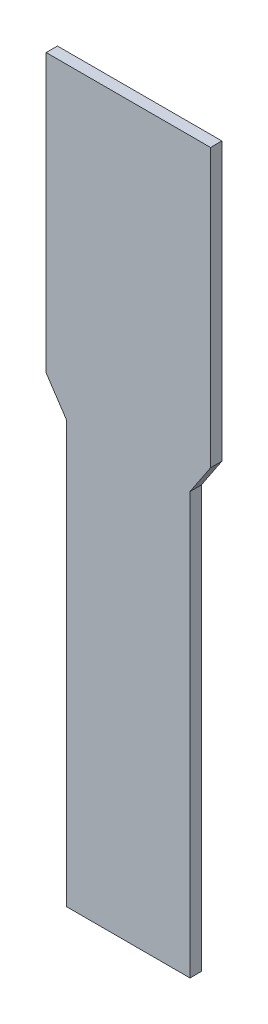
# Autodesk Inventor part: pen_type_cutter_realsize
Saved by Autodesk Inventor 2024 (Build 280153000, 153)
## iProperties
Created: 2025-06-12
Part Number: pen_type_cutter_realsize
Material: 一般
Document SubType Name: Modeling
Designer: 1412z
Density: 1 g/cm^3
Appearance: 既定
Author: 1412z
Autodesk Inventor part; units mm, degrees
ref_plane "YZ Plane" through (0, 0, 0) normal (1, 0, 0) x (0, 1, 0)
ref_plane "XZ Plane" through (0, 0, 0) normal (0, 1, 0) x (-1, 0, 0)
ref_plane "XY Plane" through (0, 0, 0) normal (0, 0, 1) x (1, 0, 0)
sketch "スケッチ1" plane through (0, 0, 0) normal (0, 0, 1) x (1, 0, 0)
  line L0 (-4, 17.75) -> (4, 17.75)
  line L1 (4, 17.75) -> (4, -17.75)
  line L2 (4, -17.75) -> (-4, -17.75)
  line L3 (-4, -17.75) -> (-4, 17.75)
  line L4 (-4, 17.75) -> (4, -17.75) construction
  line L5 (4, 17.75) -> (-4, -17.75) construction
  point P0 (0, 0)
  dimension "d0" = 8
  dimension "d1" = 35.5
  constraints: 12 end point, 2 midpoint, 2 parallel, 1 horizontal, 1 perpendicular
  measures "d0" distance of L1.end L2.end
  measures "d1" distance of L0.end L1.end
extrude "押し出し1" add sketch "スケッチ1" along normal blind 0.55
sketch "スケッチ2" plane through (0, 0, 0.55) normal (0, 0, 1) x (1, 0, 0)
  line L0 (-4, -17.75) -> (4, -17.75) projected
  line L1 (3, -17.75) -> (3, 2.75)
  line L2 (4, -17.75) -> (4, 17.75) projected
  line L3 (3, -17.75) -> (23.5, -17.75) construction
  line L4 (0, -17.75) -> (-3, -17.75)
  line L5 (-3, -17.75) -> (-3, 2.75)
  line L6 (-4, 17.75) -> (-4, -17.75) projected
  line L7 (-4, 4.25) -> (-3, 2.75)
  line L8 (-4, 4.25) -> (-4, -17.75)
  line L9 (-4, -17.75) -> (-3, -17.75)
  line L10 (4, 4.25) -> (3, 2.75)
  line L11 (4, 4.25) -> (4, -17.75)
  line L12 (3, -17.75) -> (4, -17.75)
  point P0 (0, 0)
  dimension "d4" = 20.5
  dimension "d5" = 90
  dimension "d6" = 3
  constraints: 20 end point, 5 point on line, 4 collinear, 2 perpendicular, 1 horizontal, 1 midpoint, 1 parallel
  measures "d4" distance of L1.start L1.end
  measures "d5" angle of L3 L1
  measures "d6" distance of L4.start L4.end
extrude "押し出し2" cut sketch "スケッチ2" against normal blind 0.55
